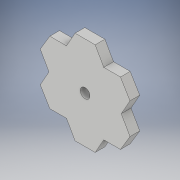
# Autodesk Inventor part: 밑판
Saved by Autodesk Inventor 2019 (Build 230136000, 136)
## iProperties
Created: 2021-07-08
Part Number: 밑판
Material: 일반
Document SubType Name: Modeling
Designer: msj19
Density: 1 g/cm^3
Appearance: 기본값
Author: msj19
Autodesk Inventor part; units mm, degrees
ref_plane "우측면도" through (0, 0, 0) normal (1, 0, 0) x (0, 1, 0)
ref_plane "평면도" through (0, 0, 0) normal (0, 1, 0) x (-1, 0, 0)
ref_plane "정면도" through (0, 0, 0) normal (0, 0, 1) x (1, 0, 0)
sketch "스케치1" plane through (0, 0, 0) normal (0, 0, 1) x (1, 0, 0)
  line L0 (0, 0) -> (184, 0)
  line L1 (184, 0) -> (112.662, 127.3848)
  line L2 (112.662, 127.3848) -> (71.338, 127.3848)
  line L3 (71.338, 127.3848) -> (0, 0)
  line L4 (0, 0) -> (19.5, -32.6152)
  line L5 (19.5, -32.6152) -> (164.5, -32.6152)
  line L6 (164.5, -32.6152) -> (184, 0)
  line L7 (0, 63.5) -> (184, 63.5)
  line L8 (19.5, 96.1152) -> (164.5, 96.1152)
  line L9 (0, 63.5) -> (71.338, -63.8848)
  line L10 (71.338, -63.8848) -> (112.662, -63.8848)
  line L11 (112.662, -63.8848) -> (184, 63.5)
  line L12 (19.5, 96.1152) -> (0, 63.5)
  line L13 (164.5, 96.1152) -> (184, 63.5)
  circle A0 centre (92, 31.1152) radius 40
  point P0 (92, -63.8848)
  dimension "d0" = 184
  dimension "d1" = 146
  dimension "d2" = 146
  dimension "d3" = 145
  dimension "d6" = 160
  dimension "d7" = 38
  dimension "d15" = 127.3848
  dimension "d16" = 184
  dimension "d17" = 63.5
  dimension "d18" = 146
  dimension "d19" = 38
  dimension "d20" = 145
  dimension "d21" = 160
  dimension "d22" = 146
  dimension "d23" = 95
  dimension "d24" = 80
  constraints: 28 end point, 4 horizontal, 3 equal length, 2 parallel, 2 vertical alignment, 1 centre point, 1 midpoint
  measures "d0" distance of L0.start L0.end
  measures "d1" distance of L2.end L0.start
  measures "d2" distance of L0.end L1.end
  measures "d3" distance of L4.end L5.end
  measures "d6" distance between parallel lines of L2 L5
  measures "d7" distance of L5.end L0.end
  measures "d15" distance between parallel lines of L0 L2
  measures "d16" distance of L7.start L7.end
  measures "d17" distance between parallel lines of L0 L7
  measures "d18" distance of L10.end L7.end
  measures "d19" distance of L8.start L7.start
  measures "d20" distance of L8.start L8.end
  measures "d21" distance between parallel lines of L8 L10
  measures "d22" distance of L7.start L9.end
  measures "d23" distance from line of L10 A0.centre
  measures "d24" diameter of A0
extrude "돌출1" add sketch "스케치1" against normal blind 20
sketch "스케치3" plane through (0, 0, 0) normal (0, 0, 1) x (1, 0, 0)
  line L0 (0, 0) -> (184, 0)
  line L1 (92, 126.8615) -> (92, -64.5501)
  circle A0 centre (92, 31.1152) radius 40
  line L2 (71.338, -63.8848) -> (112.662, -63.8848) projected
  line L3 (112.662, 127.3848) -> (71.338, 127.3848) projected
  dimension "d27" = 184
  dimension "d28" = 92
  dimension "d29" = 80
  dimension "d30" = 191.2696
  dimension "d31" = 95
  constraints: 4 end point, 1 centre point, 1 horizontal, 1 point on line, 1 vertical
  measures "d27" distance of L0.start L0.end
  measures "d28" distance from line of L0.start L1
  measures "d29" diameter of A0
  measures "d30" distance between parallel lines of L2 L3
  measures "d31" distance from line of L2 A0.centre
hole "구멍1" at (92, 31.1152, 0) direction (0, 0, -1) diameter 20 end through all
